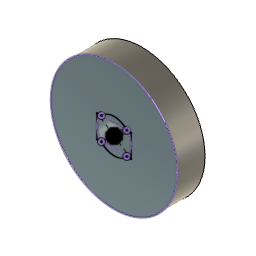
SpinningHolder v1 (Autodesk Fusion 360 design; units mm, degrees)
Autodesk Fusion 360 part; units mm, degrees
sketch "Sketch1" plane through (0, 0, 0) normal (0, 1, 0) x (1, 0, 0)
  circle A0 centre (0, 0) radius 10
  circle A1 centre (0, 0) radius 2.7
  line L0 (2.7, -1.8) -> (-2.7, -1.8)
  line L1 (-2.7, -1.8) -> (-2.7, 1.8)
  line L2 (-2.7, 1.8) -> (2.7, 1.8)
  line L3 (2.7, 1.8) -> (2.7, -1.8)
  line L4 (2.7, -1.8) -> (-2.7, 1.8) construction
  line L5 (-2.7, -1.8) -> (2.7, 1.8) construction
  dimension "d1" = 20
  dimension "d2" = 5.4
  dimension "d3" = 5.4
  dimension "d4" = 3.6
  constraint coincident A0.centre A1.centre
  constraint horizontal L0
  constraint perpendicular L0 L1
  constraint parallel L0 L2
  constraint parallel L1 L3
  constraint coincident L4 A0.centre
  constraint coincident L5 A0.centre
  measures "d1" diameter of A0
  measures "d2" diameter of A1
  measures "d3" distance of L1.end L2.end
  measures "d4" distance of L0.end L1.end
extrude "Extrude1" add sketch "Sketch1" along normal blind 4.4 contours A0 | A1 L0 L3 | A1 L2 L3 | A1 L2 | A1 L0 | A1 L1 L2 | A1 L0 L1
sketch "Sketch4" plane through (0, 0, 0) normal (0, 1, 0) x (1, 0, 0)
  arc A0 (2.0125, -1.8) -> (2.0125, 1.8) centre (0, 0) ccw
  line L0 (2.0125, 1.8) -> (-2.0125, 1.8)
  arc A1 (-2.0125, 1.8) -> (-2.0125, -1.8) centre (0, 0) ccw
  line L1 (-2.0125, -1.8) -> (2.0125, -1.8)
  circle A2 centre (0, 0) radius 10
